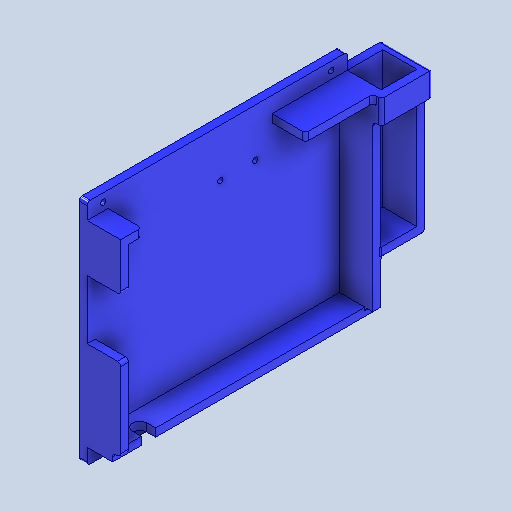
# Autodesk Inventor part: Base_v1_3DP-Pc-F
Saved by Autodesk Inventor 2025.1 (Build 291241000, 241)
## iProperties
Created: 2024-02-14
Part Number: Base_v1_3DP-Pc-F
Material: ABS プラスチック
Document SubType Name: Modeling
Designer: haruy
Density: 1.06 g/cm^3
Appearance: 青 - 壁塗料 - 光沢
Author: haruy
Autodesk Inventor part; units mm, degrees
ref_plane "YZ Plane" through (0, 0, 0) normal (1, 0, 0) x (0, 1, 0)
sketch "スケッチ2" plane through (0, 0, 0) normal (1, 0, 0) x (0, 1, 0)
  line L0 (-56.65, 76.65) -> (56.65, 76.65)
  line L1 (56.65, 76.65) -> (56.65, -76.65)
  line L2 (56.65, -76.65) -> (-56.65, -76.65)
  line L3 (-56.65, -76.65) -> (-56.65, 76.65)
  line L4 (-56.65, 76.65) -> (56.65, -76.65) construction
  line L5 (56.65, 76.65) -> (-56.65, -76.65) construction
  line L6 (61.65, -81.65) -> (61.65, 81.65)
  line L7 (61.65, 81.65) -> (-61.65, 81.65)
  line L8 (-61.65, 81.65) -> (-61.65, -81.65)
  line L9 (-61.65, -81.65) -> (61.65, -81.65)
  circle A0 centre (41.65, -1.85) radius 1.7
  circle A1 centre (41.65, -23.85) radius 1.7
  line L10 (-56.65, 76.65) -> (-56.65, 81.65)
  line L11 (-56.65, -76.65) -> (-56.65, -81.65)
  line L12 (61.65, 81.65) -> (71.65, 81.65)
  line L13 (71.65, 81.65) -> (71.65, -81.65)
  line L14 (71.65, -81.65) -> (61.65, -81.65)
  line L15 (61.65, -81.65) -> (61.65, 81.65)
  line L16 (-61.65, 81.65) -> (-71.65, 81.65)
  line L17 (-71.65, 81.65) -> (-71.65, -81.65)
  line L18 (-71.65, -81.65) -> (-61.65, -81.65)
  line L19 (-61.65, -81.65) -> (-61.65, 81.65)
  circle A2 centre (66.5, 71.5) radius 1.7
  line L20 (0, 0) -> (56.65, 0)
  line L21 (0, 0) -> (0, -76.65)
  circle A3 centre (66.5, -71.5) radius 1.7
  circle A4 centre (-66.5, 71.5) radius 1.7
  circle A5 centre (-66.5, -71.5) radius 1.7
  line L22 (61.65, -81.65) -> (-23.85, -81.65)
  line L23 (-23.85, -81.65) -> (-23.85, -103.95)
  line L24 (-23.85, -103.95) -> (61.65, -103.95)
  line L25 (61.65, -103.95) -> (61.65, -81.65)
  line L26 (61.65, -103.95) -> (-23.85, -103.95)
  line L27 (-23.85, -103.95) -> (-23.85, -108.95)
  line L28 (-23.85, -108.95) -> (61.65, -108.95)
  line L29 (61.65, -108.95) -> (61.65, -103.95)
  line L30 (-23.85, -81.65) -> (-28.85, -81.65)
  line L31 (-28.85, -81.65) -> (-28.85, -108.95)
  line L32 (-28.85, -108.95) -> (-23.85, -108.95)
  line L33 (-23.85, -108.95) -> (-23.85, -81.65)
  line L34 (61.65, -108.95) -> (46.65, -108.95)
  line L35 (46.65, -108.95) -> (46.65, -76.65)
  line L36 (46.65, -76.65) -> (61.65, -76.65)
  line L37 (61.65, -76.65) -> (61.65, -108.95)
  point P0 (-61.65, -81.65)
  point P1 (61.65, -81.65)
  point P2 (-23.85, -81.65)
  point P3 (46.65, -81.65)
  dimension "d2" = 113.3
  dimension "d3" = 153.3
  dimension "d4" = 5
  dimension "d9" = 3.4
  dimension "d10" = 3.4
  dimension "d11" = 15
  dimension "d12" = 15
  dimension "d13" = 22
  dimension "d14" = 78.5
  dimension "d45" = 10
  dimension "d46" = 163.3
  dimension "d47" = 10
  dimension "d48" = 163.3
  dimension "d49" = 3.4
  dimension "d50" = 10.15
  dimension "d51" = 5.15
  dimension "d67" = 22.3
  dimension "d68" = 85.5
  dimension "d69" = 85.5
  dimension "d70" = 5
  dimension "d71" = 5
  dimension "d72" = 27.3
  dimension "d77" = 15
  constraints: 76 end point, 16 parallel, 9 perpendicular, 7 horizontal, 6 centre point, 4 midpoint, 4 point on line, 3 symmetric about line, 6 other
  measures "d2" distance of L1.end L2.end
  measures "d3" distance of L0.end L1.end
  measures "d4" distance between parallel lines of L1 L6
  measures "d9" diameter of A0
  measures "d10" diameter of A1
  measures "d11" distance from line of A0.centre L1
  measures "d12" distance from line of A1.centre L1
  measures "d13" distance of A0.centre A1.centre
  measures "d14" distance from line of L0 A0.centre
  measures "d45" distance of L13.end L14.end
  measures "d46" distance of L12.end L13.end
  measures "d47" distance of L18.end L17.end
  measures "d48" distance of L16.end L17.end
  measures "d49" diameter of A2
  measures "d50" distance from line of L12 A2.centre
  measures "d51" distance from line of A2.centre L13
  measures "d67" distance of L24.end L14.end
  measures "d68" distance of L23.end L24.end
  measures "d69" distance of L28.end L27.end
  measures "d70" distance of L27.end L26.end
  measures "d71" distance of L32.end L31.end
  measures "d72" distance of L31.end L30.end
  measures "d77" distance of L35.end L36.end
extrude "押し出し1" add sketch "スケッチ2" along normal blind 16 contours L10 L7 L6 L36 L1 L0 | L3 L11 L9 L8 L7 L10 | L2 L35 L9 L11 | L36 L6 L9 L35 L2
extrude "押し出し2" add sketch "スケッチ2" against normal blind 5 contours L10 L7 L6 L36 L1 L0 | L0 L1 L20 L21 L2 L3 | L3 L11 L9 L8 L7 L10 | L2 L35 L9 L11 | L1 L2 L21 L20 | L36 L6 L9 L35 L2 | A0 | A1
hole "穴1" at (0, 41.65, -1.85) at (0, 41.65, -23.85) direction (-1, 0, 0) diameter 3.4 end through all
ref_plane "作業平面1" through (16, 0, 0) normal (1, 0, 0) x (0, 0, -1)
extrude "押し出し3" add sketch "スケッチ2" along normal blind 5 from surface at 16 contours L10 L7 L6 L36 L1 L0 | L2 L35 L9 L11 | L36 L6 L9 L35 L2
sketch "スケッチ3" plane through (16, -61.65, -81.65) normal (0, -1, 0) x (1, 0, 0)
  circle A0 centre (-5.5, 140.8) radius 4.5
  line L0 (0, 163.3) -> (0, 0) projected
  line L1 (-5.5, 145.3) -> (0, 145.3)
  line L2 (-5.5, 136.3) -> (0, 136.3)
  point P0 (-16, 81.65)
  point P1 (5, 158.3)
  dimension "d25" = 9
  dimension "d26" = 5.5
  dimension "d27" = 17.5
  constraints: 4 end point, 2 point on circle, 2 point on line, 2 tangent, 1 centre point, 1 parallel, 1 perpendicular
  measures "d25" diameter of A0
  measures "d26" distance from line of A0.centre L0
  measures "d27" vertical distance of point (5, 158.3) A0.centre
extrude "押し出し4" cut sketch "スケッチ3" against normal blind 5
sketch "スケッチ4" plane through (-5, -61.65, 81.65) normal (0, 0, 1) x (1, 0, 0)
  line L0 (0, 123.3) -> (26, 123.3) projected
  line L1 (26, 118.3) -> (26, 5) projected
  line L2 (0, 123.3) -> (26, 123.3)
  line L3 (26, 123.3) -> (26, 118.3)
  line L4 (26, 118.3) -> (0, 118.3)
  line L5 (0, 118.3) -> (0, 123.3)
  line L6 (0, 0) -> (21, 0) projected
  line L7 (21, 0) -> (0, 0)
  line L8 (0, 0) -> (0, 5)
  line L9 (0, 5) -> (21, 5)
  line L10 (21, 5) -> (21, 0)
  line L11 (19, 90.3) -> (13, 90.3)
  line L12 (13, 90.3) -> (13, 75.3)
  line L13 (13, 75.3) -> (19, 75.3)
  line L14 (19, 75.3) -> (19, 90.3)
  line L15 (5, 123.3) -> (5, 0)
  line L16 (0, 0) -> (0, 123.3) projected
  line L17 (17, 71.3) -> (15, 71.3)
  line L18 (15, 71.3) -> (15, 59.3)
  line L19 (15, 59.3) -> (17, 59.3)
  line L20 (17, 59.3) -> (17, 71.3)
  line L21 (22, 93.3) -> (10, 93.3)
  line L22 (10, 93.3) -> (10, 72.3)
  line L23 (10, 72.3) -> (22, 72.3)
  line L24 (22, 72.3) -> (22, 93.3)
  line L25 (20, 74.3) -> (12, 74.3)
  line L26 (12, 74.3) -> (12, 56.3)
  line L27 (12, 56.3) -> (20, 56.3)
  line L28 (20, 56.3) -> (20, 74.3)
  line L29 (20, 56.3) -> (22, 72.3)
  line L30 (12, 56.3) -> (10, 72.3)
  line L31 (22, 93.3) -> (5, 93.3)
  line L32 (22, 93.3) -> (26, 93.3)
  line L33 (12, 56.3) -> (5, 56.3)
  line L34 (26, 93.3) -> (5, 93.3)
  line L35 (5, 93.3) -> (5, 56.3)
  line L36 (5, 56.3) -> (26, 56.3)
  line L37 (26, 56.3) -> (26, 93.3)
  point P0 (5, 61.65)
  dimension "d30" = 5
  dimension "d31" = 5
  dimension "d32" = 6
  dimension "d33" = 15
  dimension "d34" = 28
  dimension "d35" = 2
  dimension "d36" = 5
  dimension "d37" = 2
  dimension "d38" = 12
  dimension "d39" = 2
  dimension "d40" = 4
  dimension "d41" = 3
  dimension "d42" = 3
  dimension "d66" = 0
  constraints: 68 end point, 14 parallel, 10 perpendicular, 6 point on line, 5 horizontal, 6 other
  measures "d30" distance of L2.end L1.start
  measures "d31" distance of L7.end L8.end
  measures "d32" distance of L13.end L12.end
  measures "d33" distance of L12.end L11.end
  measures "d34" distance between parallel lines of L4 L11
  measures "d35" distance between parallel lines of L14 L10
  measures "d36" distance between parallel lines of L15 L16
  measures "d37" distance of L19.end L18.end
  measures "d38" distance of L18.end L17.end
  measures "d39" distance between parallel lines of L12 L18
  measures "d40" distance between parallel lines of L13 L17
  measures "d41" distance between parallel lines of L14 L24
  measures "d42" distance between parallel lines of L20 L28
  measures "d66" distance from line of L33.end L15
extrude "押し出し5" cut sketch "スケッチ4" against normal blind 5 contours L31 L22 L30 L33 L15 | L1 L36 L29 L24 L32 | L21 L24 L23 L28 L25 L26 L22 | L30 L23 L26 | L26 L23 L28 L27 | L28 L23 L29 | L26 L25 L28 L23 | L14 L13 L12 L11 | L20 L19 L18 L17
sketch "スケッチ5" plane through (-5, 61.65, 81.65) normal (0, 1, 0) x (1, 0, 0)
  point P0 (5, 81.65)
extrude "押し出し6" add sketch "スケッチ2" against normal blind 5 contours L12 L13 L14 L6 | L8 L18 L17 L16
sketch "スケッチ6" plane through (21, 61.65, 81.65) normal (0, 1, 0) x (1, 0, 0)
  line L0 (-5, 32) -> (-15, 32)
  line L1 (-15, 32) -> (-15, 15)
  line L2 (-15, 15) -> (-5, 15)
  line L3 (-5, 15) -> (-5, 32)
  line L4 (-21, 163.3) -> (-21, 0) projected
  line L5 (0, 0) -> (-21, 0) projected
  line L6 (-5, 106) -> (-10.5, 106)
  line L7 (-10.5, 106) -> (-10.5, 91)
  line L8 (-10.5, 91) -> (-5, 91)
  line L9 (-5, 91) -> (-5, 106)
  line L10 (-21, 107.2) -> (-21, 103.8) projected
  line L11 (-3, 34) -> (-17, 34)
  line L12 (-17, 34) -> (-17, 13)
  line L13 (-17, 13) -> (-3, 13)
  line L14 (-3, 13) -> (-3, 34)
  line L15 (0, 0) -> (0, 163.3) projected
  line L16 (0, 116) -> (-21, 116)
  line L17 (-3, 34) -> (-3, 116)
  line L18 (-17, 34) -> (-17, 116)
  line L19 (-3, 13) -> (0, 13)
  line L20 (-17, 13) -> (-21, 13)
  line L21 (-21, 5) -> (-21, 158.3) projected
  line L22 (0, 116) -> (-21, 116)
  line L23 (-21, 116) -> (-21, 13)
  line L24 (-21, 13) -> (0, 13)
  line L25 (0, 13) -> (0, 116)
  point P0 (-21, 81.65)
  dimension "d54" = 10
  dimension "d55" = 17
  dimension "d56" = 6
  dimension "d57" = 15
  dimension "d58" = 5.5
  dimension "d59" = 15
  dimension "d60" = 10.5
  dimension "d61" = 59
  dimension "d62" = 2
  dimension "d63" = 10
  constraints: 42 end point, 9 perpendicular, 8 parallel, 6 point on line, 3 horizontal, 3 other
  measures "d54" distance of L2.end L1.end
  measures "d55" distance of L1.end L0.end
  measures "d56" distance between parallel lines of L4 L1
  measures "d57" distance between parallel lines of L2 L5
  measures "d58" distance of L8.end L7.end
  measures "d59" distance of L7.end L6.end
  measures "d60" distance between parallel lines of L10 L7
  measures "d61" distance from line of L7.end L0
  measures "d62" distance between parallel lines of L3 L14
  measures "d63" distance between parallel lines of L16 L6
extrude "押し出し7" cut sketch "スケッチ6" against normal blind 10 contours L3 L2 L1 L0 | L16 L18 L12 L20 L4 | L16 L17 L11 L18 | L16 L15 L19 L14 L17 | L11 L14 L13 L12 | L9 L8 L7 L6
extrude "押し出し8" add sketch "スケッチ2" against normal blind 5 contours L9 L23 L27 L32 L31 | L35 L24 L23 L9 | L9 L25 L24 L35 | L35 L28 L27 L24 | L24 L29 L28 L35
extrude "押し出し9" add sketch "スケッチ2" along normal blind 21.3 contours L9 L23 L27 L32 L31 | L35 L28 L27 L24 | L24 L29 L28 L35
ref_plane "作業平面2" through (21.3, 0, 0) normal (1, 0, 0) x (0, 0, -1)
extrude "押し出し10" add sketch "スケッチ2" along normal blind 5 from surface at 21.3 contours L36 L6 L9 L35 L2 | L9 L25 L24 L35 | L24 L29 L28 L35
extrude "押し出し11" add sketch "スケッチ2" against normal up to surface (0.3 mm away) from surface at 21.3 contours L36 L6 L9 L35 L2
fillet "フィレット1" radius 2 19 edges at (21, -26.35, -81.65) (21, 46.65, -79.15) (21, 59.15, -76.65) (26.3, 54.15, -76.65) (26.3, 54.15, -108.95) (16, -56.65, -79.15) (16, -56.65, 79.15) (21, -56.65, 79.15) (21, -5.35, 79.15) (21, 31.65, 79.15) (21, 59.15, -34.35) (21, 59.15, 68.65) (-2.5, 71.65, 81.65) (-2.5, 71.65, -81.65) (10.65, 61.65, -108.95) (8.15, -28.85, -108.95) (8, -28.85, -81.65) (-2.5, -71.65, -81.65) (-2.5, -71.65, 81.65)
fillet "フィレット2" radius 2 1 edges at (21.3, 46.65, -106.45)
equation "\"d12\" = d11"
